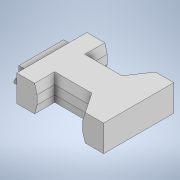
# Autodesk Inventor part: vga_plug
Saved by Autodesk Inventor 2022 (Build 260153000, 153)
## iProperties
Created: 2022-01-23
Part Number: vga_plug
Material: Generic
Document SubType Name: Modeling
Designer: kylem
Density: 1 g/cm^3
Appearance: Default
Author: kylem
Autodesk Inventor part; units mm, degrees
ref_plane "YZ Plane" through (0, 0, 0) normal (1, 0, 0) x (0, 1, 0)
ref_plane "XZ Plane" through (0, 0, 0) normal (0, 1, 0) x (-1, 0, 0)
ref_plane "XY Plane" through (0, 0, 0) normal (0, 0, 1) x (1, 0, 0)
sketch "Sketch1" plane through (0, 0, 0) normal (0, 1, 0) x (-1, 0, 0)
  line L0 (0, 0) -> (49.25, 0)
  line L1 (49.25, 0) -> (49.25, -39.75)
  line L2 (49.25, -39.75) -> (0, -39.75)
  line L3 (0, -39.75) -> (0, 0)
  line L4 (49.25, 0) -> (37.75, 0)
  line L5 (37.75, 0) -> (37.75, -10)
  line L6 (37.75, -10) -> (18.75, -10)
  line L7 (0, 0) -> (12, 0)
  line L8 (12, 0) -> (18.75, -10)
  line L9 (49.25, -19.875) -> (61.5731, -19.875)
  line L10 (37.75, -39.75) -> (37.75, -29.75)
  line L11 (37.75, -29.75) -> (18.75, -29.75)
  line L12 (12, -39.75) -> (18.75, -29.75)
  dimension "d0" = 49.25
  dimension "d1" = 39.75
  dimension "d2" = 11.5
  dimension "d3" = 10
  dimension "d4" = 19
  dimension "d5" = 12
  constraints: 26 end point, 4 symmetric about line, 3 parallel, 2 horizontal, 2 perpendicular, 2 point on line, 1 midpoint
  measures "d0" distance of L1.end L2.end
  measures "d1" distance of L0.end L1.end
  measures "d2" distance of L0.end L4.end
  measures "d3" distance of L4.end L5.end
  measures "d4" distance of L5.end L6.end
  measures "d5" distance of L0.start L7.end
extrude "Extrusion1" add sketch "Sketch1" along normal blind 15 contours L0 L8 L6 L5 L1 L2 L10 L11 L12 L3
chamfer "Chamfer1" distance 5 angle 15 1 edges at (-28.25, 15, -10) measured on face at (-31.4167, 5, -10)
chamfer "Chamfer2" distance 5 angle 15 1 edges at (-15.375, 15, -5) measured on face at (-14.25, 8.3333, -3.3333)
chamfer "Chamfer3" distance 5 angle 15 1 edges at (-37.75, 15, -5) measured on face at (-37.75, 8.3333, -3.3333)
chamfer "Chamfer4" distance 5 angle 15 1 edges at (-37.75, 0, -5) measured on face at (-37.75, 3.3333, -3.3333)
chamfer "Chamfer5" distance 5 angle 15 1 edges at (-28.25, 0, -10) measured on face at (-25.0833, 5, -10)
chamfer "Chamfer6" distance 5 angle 15 1 edges at (-15.375, 0, -5) measured on face at (-14.25, 5, -3.3333)
chamfer "Chamfer7" distance 5 angle 15 1 edges at (-28.25, 15, -29.75) measured on face at (-25.0833, 5, -29.75)
chamfer "Chamfer8" distance 5 angle 15 1 edges at (-15.375, 15, -34.75) measured on face at (-14.25, 8.3333, -36.4167)
chamfer "Chamfer9" distance 5 angle 15 1 edges at (-15.375, 0, -34.75) measured on face at (-14.25, 6.6667, -36.4167)
chamfer "Chamfer10" distance 5 angle 15 1 edges at (-28.25, 0, -29.75) measured on face at (-31.4167, 5, -29.75)
chamfer "Chamfer11" distance 5 angle 15 1 edges at (-37.75, 15, -34.75) measured on face at (-37.75, 8.3333, -36.4167)
chamfer "Chamfer12" distance 5 angle 15 1 edges at (-37.75, 0, -34.75) measured on face at (-37.75, 5.0002, -36.4167)
sketch "Sketch2" plane through (-49.25, 0, -39.75) normal (-1, 0, 0) x (0, 0, 1)
  line L0 (39.75, 0) -> (0, 0) projected
  line L1 (19.875, 0) -> (7.175, 0)
  line L2 (7.175, 0) -> (32.575, 0)
  line L3 (32.575, 0) -> (32.575, 15)
  line L4 (28.4103, 15) -> (39.75, 15) projected
  line L5 (32.575, 7.5) -> (32.575, 3)
  line L6 (32.575, 3) -> (32.575, 12)
  line L7 (7.175, 0) -> (7.175, 15)
  line L8 (32.575, 12) -> (7.175, 12)
  line L9 (7.175, 12) -> (7.175, 3)
  line L10 (7.175, 3) -> (32.575, 3)
  line L11 (32.575, 3) -> (32.575, 12)
  point P0 (7.175, 12)
  dimension "d44" = 12.7
  dimension "d45" = 25.4
  dimension "d46" = 4.5
  dimension "d47" = 9
  constraints: 20 end point, 6 point on line, 2 midpoint, 2 parallel, 2 perpendicular, 1 horizontal, 1 vertical
  measures "d44" distance of L1.start L1.end
  measures "d45" distance of L1.end L2.end
  measures "d46" distance of L5.start L5.end
  measures "d47" distance of L5.end L6.end
extrude "Extrusion2" add sketch "Sketch2" along normal blind 6 contours L10 L7 L8 L3
chamfer "Chamfer13" distance 5 angle 10 1 edges at (-52.25, 3, -32.575) measured on face at (-51.25, 9, -32.575)
chamfer "Chamfer14" distance 5 angle 10 1 edges at (-52.25, 3, -7.175) measured on face at (-51.25, 6, -7.175)
sketch "Sketch3" plane through (-49.25, 0, -39.75) normal (-1, 0, 0) x (0, 0, 1)
  line L0 (39.75, 0) -> (39.75, 15) projected
  line L1 (39.75, 7.5) -> (36.25, 7.5)
  line L2 (0, 15) -> (39.75, 15) projected
  line L3 (19.875, 15) -> (19.875, 18.5612)
  circle A0 centre (36.25, 7.5) radius 1.35
  circle A1 centre (3.5, 7.5) radius 1.35
  dimension "d56" = 3.5
  dimension "d57" = 2.7
  constraints: 4 end point, 2 centre point, 2 midpoint, 1 coincident, 1 horizontal, 1 symmetric about line, 1 vertical, 1 other
  measures "d56" distance of L1.start L1.end
  measures "d57" diameter of A0
extrude "Extrusion3" add sketch "Sketch3" along normal blind 3.8
body "Solid1"
